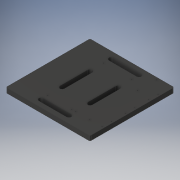
# Autodesk Inventor part: TopPlateV1
Saved by Autodesk Inventor 2017 (Build 210142000, 142)
## iProperties
Created: 2017-03-10
Part Number: TopPlateV1
Material: Polyethylene, High Density
Document SubType Name: Modeling
Designer: Naga
Density: 0.952 g/cm^3
Appearance: Smooth - Black
Author: Naga
Autodesk Inventor part; units mm, degrees
ref_plane "YZ Plane" through (0, 0, 0) normal (1, 0, 0) x (0, 1, 0)
ref_plane "XZ Plane" through (0, 0, 0) normal (0, 1, 0) x (-1, 0, 0)
ref_plane "XY Plane" through (0, 0, 0) normal (0, 0, 1) x (1, 0, 0)
sketch "Sketch1" plane through (0, 0, 0) normal (0, 1, 0) x (-1, 0, 0)
  line L0 (-114.3, 114.3) -> (114.3, 114.3)
  line L1 (114.3, 114.3) -> (114.3, -114.3)
  line L2 (114.3, -114.3) -> (-114.3, -114.3)
  line L3 (-114.3, -114.3) -> (-114.3, 114.3)
  line L4 (-114.3, 114.3) -> (114.3, -114.3) construction
  line L5 (114.3, 114.3) -> (-114.3, -114.3) construction
  line L6 (114.3, 114.3) -> (38.1, 114.3)
  line L7 (38.1, 114.3) -> (38.1, 76.2) construction
  line L8 (38.1, 76.2) -> (114.3, 76.2) construction
  line L9 (114.3, 76.2) -> (114.3, 114.3)
  circle A0 centre (38.1, 76.2) radius 1.5875
  line L10 (114.3, 0) -> (47.3217, 0)
  line L11 (-114.3, 114.3) -> (-38.1, 114.3)
  line L12 (-38.1, 114.3) -> (-38.1, 76.2) construction
  line L13 (-38.1, 76.2) -> (-114.3, 76.2) construction
  line L14 (-114.3, 76.2) -> (-114.3, 114.3)
  circle A1 centre (-38.1, 76.2) radius 1.5875
  line L15 (-114.3, -114.3) -> (-38.1, -114.3)
  line L16 (-38.1, -114.3) -> (-38.1, -76.2) construction
  line L17 (-38.1, -76.2) -> (-114.3, -76.2) construction
  line L18 (-114.3, -76.2) -> (-114.3, -114.3)
  line L19 (114.3, -114.3) -> (38.1, -114.3)
  line L20 (38.1, -114.3) -> (38.1, -76.2) construction
  line L21 (38.1, -76.2) -> (114.3, -76.2) construction
  line L22 (114.3, -76.2) -> (114.3, -114.3)
  circle A2 centre (-38.1, -76.2) radius 1.5875
  circle A3 centre (38.1, -76.2) radius 1.5875
  point P0 (0, 0)
  dimension "d0" = 228.6
  dimension "d1" = 228.6
  dimension "d2" = 76.2
  dimension "d3" = 38.1
  dimension "d4" = 3.175
  dimension "d5" = 76.2
  dimension "d6" = 3.175
  dimension "d7" = 38.1
  dimension "d8" = 76.2
  dimension "d9" = 3.175
  dimension "d10" = 3.175
  constraints: 46 end point, 10 parallel, 6 horizontal, 5 perpendicular, 4 centre point, 4 coincident, 3 midpoint
  measures "d0" distance of L1.end L2.end
  measures "d1" distance of L0.end L1.end
  measures "d2" distance of L8.end L7.end
  measures "d3" distance of L7.end L6.end
  measures "d4" diameter of A0
  measures "d5" distance of L12.end L13.end
  measures "d6" diameter of A1
  measures "d7" distance of L16.end L15.end
  measures "d8" distance of L20.end L21.end
  measures "d9" diameter of A2
  measures "d10" diameter of A3
extrude "Extrusion1" add sketch "Sketch1" along normal blind 12.7
fillet "Fillet1" radius 3.175 4 edges at (-114.3, 6.35, 114.3) (114.3, 6.35, 114.3) (114.3, 6.35, -114.3) (-114.3, 6.35, -114.3)
sketch "Sketch4" plane through (0, 12.7, 0) normal (0, 1, 0) x (1, 0, 0)
  circle A0 centre (-38.1, 76.2) radius 1.5875 projected
  circle A1 centre (38.1, 76.2) radius 1.5875 projected
  circle A2 centre (38.1, -76.2) radius 1.5875 projected
  circle A3 centre (-38.1, -76.2) radius 1.5875 projected
  arc A4 (-111.125, 114.3) -> (-114.3, 111.125) centre (-111.125, 111.125) ccw projected
  line L0 (-114.3, 111.125) -> (-114.3, -111.125) projected
  arc A5 (-114.3, -111.125) -> (-111.125, -114.3) centre (-111.125, -111.125) ccw projected
  line L1 (-111.125, -114.3) -> (111.125, -114.3) projected
  arc A6 (111.125, -114.3) -> (114.3, -111.125) centre (111.125, -111.125) ccw projected
  line L2 (114.3, -111.125) -> (114.3, 111.125) projected
  arc A7 (114.3, 111.125) -> (111.125, 114.3) centre (111.125, 111.125) ccw projected
  line L3 (111.125, 114.3) -> (-111.125, 114.3) projected
  line L4 (114.3, 114.3) -> (73.025, 114.3) construction
  line L5 (73.025, 114.3) -> (73.025, 107.95) construction
  line L6 (73.025, 107.95) -> (114.3, 107.95) construction
  line L7 (114.3, 107.95) -> (114.3, 114.3) construction
  line L8 (114.3, 114.3) -> (73.025, 114.3) construction
  line L9 (73.025, 114.3) -> (73.025, 57.15) construction
  line L10 (73.025, 57.15) -> (114.3, 57.15) construction
  line L11 (114.3, 57.15) -> (114.3, 114.3) construction
  circle A8 centre (73.025, 57.15) radius 1.5875
  circle A9 centre (73.025, 107.95) radius 1.5875
  point P0 (0, 0)
  dimension "d22" = 41.275
  dimension "d23" = 6.35
  dimension "d24" = 57.15
  dimension "d25" = 3.175
  dimension "d26" = 3.175
  constraints: 16 end point, 4 parallel, 2 centre point, 2 coincident, 2 horizontal, 2 perpendicular, 1 point on line
  measures "d22" distance of L6.end L5.end
  measures "d23" distance of L5.end L4.end
  measures "d24" distance of L9.end L8.end
  measures "d25" diameter of A8
  measures "d26" diameter of A9
extrude "camMount" cut sketch "Sketch4" against normal up to surface (12.7 mm away) contours A8 | A9
sketch "Sketch5" plane through (0, 12.7, 0) normal (0, 1, 0) x (1, 0, 0)
  circle A0 centre (73.025, 57.15) radius 1.5875 construction
  circle A1 centre (73.025, 107.95) radius 1.5875 construction
  circle A2 centre (-38.1, 76.2) radius 1.5875 construction
  circle A3 centre (38.1, 76.2) radius 1.5875 construction
  circle A4 centre (38.1, -76.2) radius 1.5875 construction
  circle A5 centre (-38.1, -76.2) radius 1.5875 construction
  arc A6 (-111.125, 114.3) -> (-114.3, 111.125) centre (-111.125, 111.125) ccw construction
  line L0 (-114.3, 111.125) -> (-114.3, -111.125) construction
  arc A7 (-114.3, -111.125) -> (-111.125, -114.3) centre (-111.125, -111.125) ccw construction
  line L1 (-111.125, -114.3) -> (111.125, -114.3) construction
  arc A8 (111.125, -114.3) -> (114.3, -111.125) centre (111.125, -111.125) ccw construction
  line L2 (114.3, -111.125) -> (114.3, 111.125) construction
  arc A9 (114.3, 111.125) -> (111.125, 114.3) centre (111.125, 111.125) ccw construction
  line L3 (111.125, 114.3) -> (-111.125, 114.3) construction
  line L4 (114.3, -114.3) -> (107.95, -114.3) construction
  line L5 (107.95, -77.089) -> (114.3, -77.089) construction
  line L6 (114.3, -77.089) -> (114.3, -114.3) construction
  line L7 (114.3, -114.3) -> (59.6392, -114.3) construction
  line L8 (59.6392, -77.089) -> (114.3, -77.089) construction
  line L9 (114.3, -77.089) -> (114.3, -114.3) construction
  line L10 (114.3, -114.3) -> (27.8892, -114.3) construction
  line L11 (27.8892, -114.3) -> (27.8892, -77.089) construction
  line L12 (27.8892, -77.089) -> (114.3, -77.089) construction
  line L13 (114.3, -77.089) -> (114.3, -114.3) construction
  line L14 (114.3, -114.3) -> (76.2, -114.3) construction
  line L15 (76.2, -114.3) -> (76.2, -77.089) construction
  line L16 (76.2, -77.089) -> (114.3, -77.089) construction
  line L17 (114.3, -77.089) -> (114.3, -114.3) construction
  circle A10 centre (76.2, -77.089) radius 1.5875 construction
  circle A11 centre (76.2, -77.089) radius 1.5875
  circle A12 centre (27.8892, -77.089) radius 1.5875
  point P0 (0, 0)
  dimension "d29" = 6.35
  dimension "d30" = 37.211
  dimension "d31" = 54.6608
  dimension "d36" = 86.4108
  dimension "d37" = 38.1
  dimension "d38" = 3.175
  constraints: 28 end point, 6 parallel, 4 horizontal, 3 centre point, 3 coincident, 2 perpendicular, 2 point on line, 1 concentric
  measures "d29" distance of L5.start L5.end
  measures "d30" distance of L4.end L5.start
  measures "d31" distance of L8.start L8.end
  measures "d36" distance of L11.end L12.end
  measures "d37" distance of L15.end L16.end
  measures "d38" diameter of A10
extrude "TilitMount" cut sketch "Sketch5" against normal up to surface (12.7 mm away)
sketch "Sketch6" plane through (0, 12.7, 0) normal (0, 1, 0) x (1, 0, 0)
  line L0 (38.1, -95.25) -> (-38.1, -95.25)
  line L1 (-38.1, -95.25) -> (-38.1, 95.25)
  line L2 (-38.1, 95.25) -> (38.1, 95.25)
  line L3 (38.1, 95.25) -> (38.1, -95.25)
  line L4 (38.1, -95.25) -> (-38.1, 95.25) construction
  line L5 (-38.1, -95.25) -> (38.1, 95.25) construction
  line L6 (-38.1, -95.25) -> (38.1, -95.25) construction
  line L7 (-38.1, -101.6) -> (38.1, -101.6)
  line L8 (38.1, -88.9) -> (-38.1, -88.9)
  arc A0 (-38.1, -88.9) -> (-38.1, -101.6) centre (-38.1, -95.25) ccw
  arc A1 (38.1, -101.6) -> (38.1, -88.9) centre (38.1, -95.25) ccw
  line L9 (-38.1, 95.25) -> (38.1, 95.25) construction
  line L10 (-38.1, 88.9) -> (38.1, 88.9)
  line L11 (38.1, 101.6) -> (-38.1, 101.6)
  arc A2 (-38.1, 101.6) -> (-38.1, 88.9) centre (-38.1, 95.25) ccw
  arc A3 (38.1, 88.9) -> (38.1, 101.6) centre (38.1, 95.25) ccw
  line L12 (38.1, -38.1) -> (-38.1, -38.1)
  line L13 (-38.1, -38.1) -> (-38.1, 38.1)
  line L14 (-38.1, 38.1) -> (38.1, 38.1)
  line L15 (38.1, 38.1) -> (38.1, -38.1)
  line L16 (38.1, -38.1) -> (-38.1, 38.1) construction
  line L17 (-38.1, -38.1) -> (38.1, 38.1) construction
  line L18 (38.1, -38.1) -> (38.1, 38.1) construction
  line L19 (44.45, -38.1) -> (44.45, 38.1)
  line L20 (31.75, 38.1) -> (31.75, -38.1)
  arc A4 (31.75, -38.1) -> (44.45, -38.1) centre (38.1, -38.1) ccw
  arc A5 (44.45, 38.1) -> (31.75, 38.1) centre (38.1, 38.1) ccw
  line L21 (-38.1, -38.1) -> (-38.1, 38.1) construction
  line L22 (-31.75, -38.1) -> (-31.75, 38.1)
  line L23 (-44.45, 38.1) -> (-44.45, -38.1)
  arc A6 (-44.45, -38.1) -> (-31.75, -38.1) centre (-38.1, -38.1) ccw
  arc A7 (-31.75, 38.1) -> (-44.45, 38.1) centre (-38.1, 38.1) ccw
  point P0 (0, 0)
  point P1 (0, -95.25)
  point P2 (0, 95.25)
  point P3 (38.1, 0)
  point P4 (-38.1, 0)
  dimension "d39" = 76.2
  dimension "d40" = 190.5
  dimension "d41" = 12.7
  dimension "d42" = 12.7
  dimension "d43" = 76.2
  dimension "d44" = 12.7
  dimension "d45" = 12.7
  constraints: 56 end point, 16 point on circle, 16 tangent, 8 centre point, 8 midpoint, 8 parallel, 4 collinear, 2 horizontal, 2 perpendicular, 1 point on line
  measures "d39" distance of L1.end L2.end
  measures "d40" distance of L0.end L1.end
  measures "d41" diameter of A1
  measures "d42" diameter of A3
  measures "d43" distance of L12.end L13.end
  measures "d44" diameter of A5
  measures "d45" diameter of A7
extrude "Extrusion6" cut sketch "Sketch6" against normal blind 25.4 contours L3 A1 L7 A0 L1 L0 | L0 L1 L8 L3 | A4 L12 L3 | L3 A5 L19 A4 | A6 L23 A7 L1 | L1 L12 A6 | L12 L20 L14 L3 | L1 L14 L22 L12 | L14 A5 L3 | L1 A7 L14 | L10 L1 L2 L3 | L3 L2 L1 A2 L11 A3
sketch "Sketch7" plane through (0, 12.7, 0) normal (0, 1, 0) x (1, 0, 0)
  line L0 (114.3, -111.125) -> (114.3, 111.125) projected
  line L1 (114.3, 0) -> (104.775, 0)
  line L2 (109.5375, 0) -> (109.5375, 12.7)
  circle A0 centre (109.5375, 12.7) radius 1.5875
  circle A1 centre (109.5375, -12.7) radius 1.5875
  point P0 (0, 0)
  dimension "d48" = 9.525
  dimension "d49" = 12.7
  dimension "d50" = 3.175
  constraints: 4 end point, 2 centre point, 2 midpoint, 1 coincident, 1 horizontal, 1 symmetric about line, 1 vertical, 1 other
  measures "d48" distance of L1.start L1.end
  measures "d49" distance of L2.start L2.end
  measures "d50" diameter of A0
extrude "Extrusion7" cut sketch "Sketch7" against normal blind 25.4
sketch "Sketch8" plane through (0, 12.7, 0) normal (0, 1, 0) x (1, 0, 0)
  circle A0 centre (109.5375, -12.7) radius 1.5875 projected
  circle A1 centre (109.5375, -12.7) radius 1.5875 construction
  line L0 (109.5375, -12.7) -> (109.5375, -50.8) construction
  line L1 (109.5375, -50.8) -> (109.5375, -76.2) construction
  circle A2 centre (109.5375, -50.8) radius 1.5875
  circle A3 centre (109.5375, -76.2) radius 1.5875
  line L2 (114.3, 111.125) -> (114.3, -111.125) projected
  line L3 (114.3, 0) -> (96.6606, 0)
  circle A4 centre (109.5375, 50.8) radius 1.5875
  circle A5 centre (109.5375, 76.2) radius 1.5875
  point P0 (0, 0)
  dimension "d53" = 38.1
  dimension "d54" = 25.4
  dimension "d55" = 3.175
  dimension "d56" = 3.175
  constraints: 6 end point, 4 centre point, 2 coincident, 2 symmetric about line, 2 vertical, 1 horizontal, 1 midpoint, 2 other
  measures "d53" distance of L0.start L0.end
  measures "d54" distance of L0.end L1.end
  measures "d55" diameter of A2
  measures "d56" diameter of A3
extrude "Extrusion8" cut sketch "Sketch8" against normal blind 25.4 contours A2 | A3 | A4 | A5
body "Solid1"
